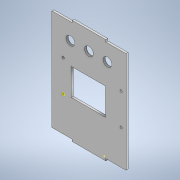
# Autodesk Inventor part: test
Saved by Autodesk Inventor 2020 (Build 240168000, 168)
## iProperties
Created: 2020-05-21
Part Number: test
Material: Generic
Document SubType Name: Modeling
Designer: jelte
Density: 1 g/cm^3
Appearance: Default
Author: jelte
Autodesk Inventor part; units mm, degrees
ref_plane "YZ Plane" through (0, 0, 0) normal (1, 0, 0) x (0, 1, 0)
ref_plane "XZ Plane" through (0, 0, 0) normal (0, 1, 0) x (-1, 0, 0)
ref_plane "XY Plane" through (0, 0, 0) normal (0, 0, 1) x (1, 0, 0)
sketch "Sketch1" plane through (0, 0, 0) normal (0, 0, 1) x (1, 0, 0)
  line L0 (-77.994, -2.3973) -> (-47.994, -2.3973)
  line L1 (-47.994, -2.3973) -> (-47.994, -5.3973)
  line L2 (-47.994, -5.3973) -> (2.006, -5.3973)
  line L3 (2.006, -2.3973) -> (32.006, -2.3973)
  line L4 (32.006, -2.3973) -> (32.006, 147.6027)
  line L5 (32.006, 147.6027) -> (2.006, 147.6027)
  line L6 (2.006, 147.6027) -> (2.006, 150.6027)
  line L7 (2.006, 150.6027) -> (-47.994, 150.6027)
  line L8 (-47.994, 150.6027) -> (-47.994, 147.6027)
  line L9 (-47.994, 147.6027) -> (-77.994, 147.6027)
  line L10 (2.006, -2.3973) -> (2.006, -5.3973)
  line L11 (-77.994, 147.6027) -> (-77.994, -2.3973)
  point P0 (0, 0)
  dimension "d0" = 150
  dimension "d1" = 3
  dimension "d2" = 3
  dimension "d3" = 50
  dimension "d4" = 50
  dimension "d5" = 30
  dimension "d6" = 30
  constraints: 24 end point, 6 perpendicular, 6 point on line, 1 parallel, 1 vertical
  measures "d0" distance of L3.end L4.end
  measures "d1" distance of L5.end L6.end
  measures "d2" distance of L3.start L2.end
  measures "d3" distance of L6.end L7.end
  measures "d4" distance of L1.end L2.end
  measures "d5" distance of L0.start L0.end
  measures "d6" distance of L3.start L3.end
extrude "Extrusion1" add sketch "Sketch1" along normal blind 3
sketch "Sketch2" plane through (0, 0, 3) normal (0, 0, 1) x (1, 0, 0)
  line L0 (27.506, 96.0027) -> (27.506, 98.7027)
  line L1 (-77.994, 147.6027) -> (-77.994, -2.3973) projected
  circle A0 centre (24.806, 49.2027) radius 1.75
  circle A1 centre (24.806, 96.0027) radius 1.75
  circle A2 centre (-61.194, 96.0027) radius 1.75
  circle A3 centre (-61.194, 49.2027) radius 1.75
  line L2 (27.506, 50.6827) -> (27.506, 46.5027)
  line L3 (1.606, 50.6827) -> (-49.394, 50.6827)
  line L4 (-49.394, 50.6827) -> (-49.394, 90.6827)
  line L5 (-49.394, 90.6827) -> (1.606, 90.6827)
  line L6 (1.606, 90.6827) -> (1.606, 50.6827)
  line L7 (32.006, 147.6027) -> (2.006, 147.6027) projected
  point P0 (0, 0)
  constraints: 12 end point, 4 centre point, 2 parallel, 1 horizontal, 1 perpendicular
extrude "Extrusion2" cut sketch "Sketch2" against normal blind 3
sketch "Sketch3" plane through (0, 0, 3) normal (0, 0, 1) x (1, 0, 0)
  circle A0 centre (-61.194, 49.2027) radius 1.75 projected
  point P0 (0, 0)
sketch "Sketch4" plane through (0, 0, 3) normal (0, 0, 1) x (1, 0, 0)
  circle A0 centre (-61.194, 96.0027) radius 1.75 projected
  line L0 (-77.994, 147.6027) -> (-77.994, -2.3973) projected
  circle A1 centre (-50.494, 123.146) radius 6.5
  circle A2 centre (-22.994, 123.146) radius 6.5
  circle A3 centre (4.506, 123.146) radius 6.5
  point P0 (0, 0)
  point P1 (32.006, 147.6027)
  dimension "d48" = 13
  dimension "d49" = 13
  dimension "d50" = 13
  constraints: 3 centre point
  measures "d48" diameter of A3
  measures "d49" diameter of A2
  measures "d50" diameter of A1
extrude "Extrusion3" cut sketch "Sketch4" against normal blind 3 contours A1 | A2 | A3
body "Solid1"
